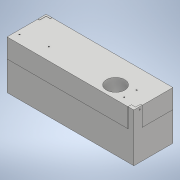
# Autodesk Inventor part: 1руб
Saved by Autodesk Inventor 2020 (Build 240168000, 168)
## iProperties
Created: 2020-02-01
Part Number: 1руб
Material: Типовые
Document SubType Name: Modeling
Designer: Css38
Density: 1 g/cm^3
Appearance: По умолчанию
Author: Css38
Autodesk Inventor part; units mm, degrees
ref_plane "YZ Plane" through (0, 0, 0) normal (1, 0, 0) x (0, 1, 0)
ref_plane "XZ Plane" through (0, 0, 0) normal (0, 1, 0) x (-1, 0, 0)
sketch "Эскиз1" plane through (0, 0, 0) normal (0, 0, 1) x (1, 0, 0)
  line L0 (-76.25, 23.5) -> (76.25, 23.5)
  line L1 (76.25, 23.5) -> (76.25, -23.5)
  line L2 (76.25, -23.5) -> (-76.25, -23.5)
  line L3 (-76.25, -23.5) -> (-76.25, 23.5)
  line L4 (-76.25, 23.5) -> (76.25, -23.5) construction
  line L5 (76.25, 23.5) -> (-76.25, -23.5) construction
  point P0 (0, 0)
  point P1 (0, 0)
  dimension "d35" = 152.5
  dimension "d36" = 47
  constraints: 12 end point, 2 parallel, 1 coincident, 1 horizontal, 1 midpoint, 1 perpendicular
  measures "d35" distance of L1.end L2.end
  measures "d36" distance of L2.end L0.start
extrude "Выдавливание1" add sketch "Эскиз1" along normal blind 30
sketch "Эскиз2" plane through (0, 0, 30) normal (0, 0, 1) x (1, 0, 0)
  line L0 (76.25, 23.5) -> (76.25, -23.5) construction
  line L1 (76.25, -23.5) -> (-76.25, -23.5) construction
  line L2 (-76.25, -23.5) -> (-76.25, 23.5) construction
  line L3 (-76.25, 23.5) -> (76.25, 23.5) construction
  line L4 (74.25, -19.5) -> (51.75, -19.5)
  line L5 (51.75, -19.5) -> (51.75, 3)
  line L6 (51.75, 3) -> (74.25, 3)
  line L7 (74.25, 3) -> (74.25, -19.5)
  point P0 (0, 0)
  dimension "d40" = 22.5
  dimension "d142" = 2
  dimension "d143" = 4
  constraints: 8 end point, 2 parallel, 2 perpendicular, 1 horizontal
  measures "d40" distance of L5.end L6.end
  measures "d142" distance between parallel lines of L0 L7
  measures "d143" distance between parallel lines of L1 L4
extrude "Выдавливание2" cut sketch "Эскиз2" against normal up to next
sketch "Эскиз3" plane through (0, 0, 30) normal (0, 0, 1) x (1, 0, 0)
  line L0 (51.75, 3) -> (51.75, -19.5)
  line L1 (51.75, -19.5) -> (74.25, -19.5)
  line L2 (74.25, -19.5) -> (74.25, 3)
  line L3 (74.25, 3) -> (51.75, 3)
  line L4 (76.25, 23.5) -> (76.25, -23.5) construction
  line L5 (76.25, -23.5) -> (-76.25, -23.5) construction
  line L6 (-76.25, 23.5) -> (76.25, 23.5) construction
  line L7 (76.25, 23.5) -> (-76.25, 23.5) projected
  line L8 (-76.25, 23.5) -> (76.25, 23.5)
  line L9 (76.25, 23.5) -> (76.25, -23.5)
  line L10 (76.25, -23.5) -> (-76.25, -23.5)
  line L11 (-76.25, 23.5) -> (-76.25, 21.5)
  line L12 (-76.25, 23.5) -> (-76.25, -23.5) construction
  line L13 (-76.25, 21.5) -> (6.25, 21.5)
  line L14 (6.25, 21.5) -> (6.25, 3)
  line L15 (6.25, 3) -> (26.25, 3)
  line L16 (26.25, 3) -> (26.25, -19.5)
  line L17 (26.25, -19.5) -> (-76.25, -19.5)
  line L18 (-76.25, -23.5) -> (-76.25, -19.5)
  line L19 (-76.25, -23.5) -> (76.25, -23.5) projected
  line L20 (76.25, -23.5) -> (76.25, 23.5) projected
  line L21 (74.25, -19.5) -> (51.75, -19.5) projected
  line L22 (51.75, -19.5) -> (51.75, 3) projected
  line L23 (51.75, 3) -> (74.25, 3) projected
  line L24 (74.25, 3) -> (74.25, -19.5) projected
  dimension "d50" = 2
  dimension "d63" = 25.5
  dimension "d130" = 20
  constraints: 34 end point, 13 collinear, 4 perpendicular, 2 parallel, 2 point on line
  measures "d50" distance of L6.start L11.end
  measures "d63" distance between parallel lines of L0 L16
  measures "d130" distance of L14.end L15.end
extrude "Выдавливание4" add sketch "Эскиз3" along normal blind 3
sketch "Эскиз4" plane through (0, 0, 33) normal (0, 0, 1) x (1, 0, 0)
  line L0 (51.75, 3) -> (51.75, -19.5) construction
  line L1 (51.75, -19.5) -> (74.25, -19.5) construction
  line L2 (74.25, -19.5) -> (74.25, 3) construction
  line L3 (74.25, 3) -> (51.75, 3) construction
  line L4 (76.25, 23.5) -> (76.25, -23.5) projected
  line L5 (76.25, -23.5) -> (-76.25, -23.5) projected
  line L6 (-76.25, -23.5) -> (-76.25, -19.5) projected
  line L7 (-76.25, -19.5) -> (26.25, -19.5) projected
  line L8 (26.25, -19.5) -> (26.25, 3) projected
  line L9 (26.25, 3) -> (6.25, 3) projected
  line L10 (6.25, 3) -> (6.25, 21.5) projected
  line L11 (6.25, 21.5) -> (-76.25, 21.5) projected
  line L12 (-76.25, 21.5) -> (-76.25, 23.5) projected
  line L13 (-76.25, 23.5) -> (76.25, 23.5) projected
  line L14 (26.25, -19.5) -> (26.25, 3) projected
  line L15 (26.25, 3) -> (51.75, 3) construction
  line L16 (51.75, 3) -> (51.75, -19.5) projected
  line L17 (51.75, -19.5) -> (26.25, -19.5) construction
  circle A0 centre (39, -8.25) radius 11
  line L18 (39, -8.25) -> (39, 3) construction
  line L19 (39, -8.25) -> (39, -19.5) construction
  line L20 (51.75, -19.5) -> (51.75, 3) construction
  line L21 (39, -8.25) -> (26.25, -8.25) construction
  line L22 (39, -8.25) -> (51.75, -8.25) construction
  point P0 (0, 0)
  dimension "d55" = 22
  constraints: 12 end point, 4 midpoint, 3 perpendicular, 2 collinear, 1 centre point, 1 point on line, 1 other
  measures "d55" diameter of A0
extrude "Выдавливание7" add sketch "Эскиз4" along normal blind 25
sketch "Эскиз6" plane through (26.25, -19.5, 30) normal (-1, 0, 0) x (0, 0, 1)
  line L0 (3, 0.25) -> (3, 22.25) construction
  line L1 (0, 22.5) -> (28, 22.5) projected
  line L2 (0, 0) -> (28, 0) projected
  line L3 (3, 22.5) -> (5, 22.5)
  line L4 (5, 22.5) -> (5, 0)
  line L5 (5, 0) -> (3, 0)
  line L6 (3, 0) -> (3, 22.5)
  point P0 (-30, 19.5)
  dimension "d66" = 2
  constraints: 8 end point, 2 parallel, 2 point on line, 1 collinear, 1 horizontal, 1 perpendicular
  measures "d66" distance of L4.end L5.end
extrude "Выдавливание8" cut sketch "Эскиз6" against normal up to surface (48 mm away) from surface at 0
sketch "Эскиз7" plane through (0, 0, 58) normal (0, 0, 1) x (1, 0, 0)
  line L0 (76.25, -23.5) -> (-76.25, -23.5) projected
  line L1 (-76.25, 23.5) -> (76.25, 23.5) projected
  line L2 (76.25, -23.5) -> (-76.25, -23.5)
  line L3 (-76.25, -23.5) -> (-76.25, 23.5)
  line L4 (-76.25, 23.5) -> (76.25, 23.5)
  line L5 (76.25, 23.5) -> (76.25, -23.5)
  circle A0 centre (39, -8.25) radius 11 projected
  point P0 (0, 0)
  constraints: 8 end point, 2 parallel, 1 horizontal, 1 perpendicular
extrude "Выдавливание9" add sketch "Эскиз7" against normal blind 17.15
ref_plane "РабПлоскость1" through (26.25, 3, 35) normal (0, 0, -1) x (-1, 0, 0)
split body "Разделение1" result two bodies by plane through (26.25, 3, 35) normal (0, 0, -1) first body at (-33.5833, 1, 0.5)
sketch "Эскиз22" plane through (0, 0, 30) normal (0, 0, 1) x (1, 0, 0)
  line L0 (-76.25, -19.5) -> (26.25, -19.5) construction
  line L1 (26.25, -19.5) -> (26.25, 3) construction
  line L2 (26.25, 3) -> (6.25, 3) construction
  line L3 (6.25, 3) -> (6.25, 21.5) construction
  line L4 (6.25, 21.5) -> (-76.25, 21.5) construction
  line L5 (-76.25, -19.5) -> (-76.25, 21.5) construction
  line L6 (-76.25, -23.5) -> (-76.25, -19.5) construction
  line L7 (76.25, -23.5) -> (-76.25, -23.5) construction
  line L8 (76.25, 23.5) -> (76.25, -23.5) construction
  line L9 (-76.25, 23.5) -> (76.25, 23.5) construction
  line L10 (74.25, 3) -> (51.75, 3) construction
  line L11 (51.75, 3) -> (51.75, -19.5) construction
  line L12 (51.75, -19.5) -> (74.25, -19.5) construction
  line L13 (74.25, -19.5) -> (74.25, 3) construction
  line L14 (-76.25, -19.5) -> (-43.25, -19.5)
  line L15 (-43.25, -19.5) -> (-43.25, -7)
  line L16 (-43.25, -7) -> (-76.25, -7)
  line L17 (-76.25, -7) -> (-76.25, -19.5)
  line L18 (-76.25, 21.5) -> (-76.25, 23.5) projected
  point P0 (0, 0)
  dimension "d144" = 33
  dimension "d145" = 12.5
  constraints: 8 end point, 2 parallel, 1 horizontal, 1 perpendicular
  measures "d144" distance of L16.end L15.end
  measures "d145" distance of L15.end L14.end
extrude "Выдавливание26" cut sketch "Эскиз22" against normal blind 28 bodies 2
sketch "Эскиз23" plane through (0, 0, 2) normal (0, 0, 1) x (1, 0, 0)
  line L0 (76.25, 23.5) -> (76.25, -23.5) construction
  line L1 (76.25, -23.5) -> (-76.25, -23.5) construction
  line L2 (-76.25, -23.5) -> (-76.25, -19.5) construction
  line L3 (-76.25, -19.5) -> (-76.25, -7) construction
  line L4 (-43.25, -7) -> (-76.25, -7) construction
  line L5 (-43.25, -19.5) -> (-43.25, -7) construction
  line L6 (-76.25, -19.5) -> (-43.25, -19.5) construction
  line L7 (-76.25, 23.5) -> (76.25, 23.5) construction
  line L8 (-76.25, -7) -> (-76.25, 23.5) construction
  line L9 (74.25, 3) -> (51.75, 3) construction
  line L10 (51.75, 3) -> (51.75, -19.5) construction
  line L11 (51.75, -19.5) -> (74.25, -19.5) construction
  line L12 (74.25, -19.5) -> (74.25, 3) construction
  line L13 (-43.25, -19.5) -> (-47.75, -19.5)
  line L14 (-47.75, -19.5) -> (-47.75, -7)
  line L15 (-47.75, -7) -> (-43.25, -7)
  line L16 (-43.25, -7) -> (-43.25, -19.5)
  point P0 (0, 0)
  dimension "d148" = 4.5
  constraints: 8 end point, 2 parallel, 1 horizontal, 1 perpendicular, 1 point on line
  measures "d148" distance of L14.end L15.end
extrude "Выдавливание27" add sketch "Эскиз23" along normal blind 18 bodies 2
sketch "Эскиз24" plane through (0, 0, 20) normal (0, 0, 1) x (1, 0, 0)
  line L0 (76.25, 23.5) -> (76.25, -23.5) construction
  line L1 (76.25, -23.5) -> (-76.25, -23.5) construction
  line L2 (-76.25, -23.5) -> (-76.25, -19.5) construction
  line L3 (-76.25, -19.5) -> (-47.75, -19.5) construction
  line L4 (-47.75, -19.5) -> (-47.75, -7) construction
  line L5 (-43.25, -7) -> (-47.75, -7) construction
  line L6 (-43.25, -19.5) -> (-43.25, -7) construction
  line L7 (-47.75, -19.5) -> (-43.25, -19.5) construction
  line L8 (-76.25, 23.5) -> (76.25, 23.5) construction
  line L9 (-76.25, -7) -> (-76.25, 23.5) construction
  line L10 (-47.75, -7) -> (-76.25, -7) construction
  line L11 (74.25, 3) -> (51.75, 3) construction
  line L12 (51.75, 3) -> (51.75, -19.5) construction
  line L13 (51.75, -19.5) -> (74.25, -19.5) construction
  line L14 (74.25, -19.5) -> (74.25, 3) construction
  line L15 (-76.25, -7) -> (-47.75, -7) construction
  line L16 (-43.25, -19.5) -> (-47.75, -7) construction
  line L17 (-47.75, -19.5) -> (-47.75, -7) construction
  line L18 (-47.75, -7) -> (-47.75, -19.5) construction
  line L19 (-47.75, -19.5) -> (-43.25, -7) construction
  circle A0 centre (-45.5, -13.25) radius 0.75
  point P0 (0, 0)
  dimension "d151" = 1.5
  constraints: 6 end point, 1 centre point, 1 collinear, 1 midpoint
  measures "d151" diameter of A0
extrude "Выдавливание28" cut sketch "Эскиз24" against normal blind 3 bodies 2
sketch "Эскиз25" plane through (0, 0, 30) normal (0, 0, 1) x (1, 0, 0)
  line L0 (76.25, 23.5) -> (76.25, -23.5) construction
  line L1 (76.25, -23.5) -> (-76.25, -23.5) construction
  line L2 (-76.25, -23.5) -> (-76.25, -19.5) construction
  line L3 (-76.25, -19.5) -> (-43.25, -19.5) construction
  line L4 (-43.25, -19.5) -> (26.25, -19.5) construction
  line L5 (26.25, -19.5) -> (26.25, 3) construction
  line L6 (26.25, 3) -> (6.25, 3) construction
  line L7 (6.25, 3) -> (6.25, 21.5) construction
  line L8 (6.25, 21.5) -> (-76.25, 21.5) construction
  line L9 (-76.25, -7) -> (-76.25, 21.5) construction
  line L10 (-43.25, -7) -> (-76.25, -7) construction
  line L11 (-43.25, -19.5) -> (-43.25, -7) construction
  line L12 (-76.25, 23.5) -> (76.25, 23.5) construction
  line L13 (74.25, 3) -> (51.75, 3) construction
  line L14 (51.75, 3) -> (51.75, -19.5) construction
  line L15 (51.75, -19.5) -> (74.25, -19.5) construction
  line L16 (74.25, -19.5) -> (74.25, 3) construction
  line L17 (-76.25, -19.5) -> (-76.25, -7) construction
  line L18 (51.75, 3) -> (51.75, -19.5) construction
  line L19 (27.3887, -8.25) -> (-21.6113, -8.25)
  line L20 (-65.25, -13.25) -> (-45.6782, 15.7663)
  line L21 (-43.25, -7) -> (-43.25, -19.5) construction
  line L22 (-45.6782, 15.7663) -> (-21.6113, -8.25)
  line L23 (-76.25, 21.5) -> (-76.25, 23.5) projected
  point P0 (0, 0)
  point P1 (-43.25, -13.25)
  point P2 (51.75, -8.25)
  dimension "d154" = 11
  dimension "d155" = 49
  dimension "d156" = 35
  dimension "d159" = 34
  dimension "d164" = 56
  constraints: 6 end point, 2 midpoint, 1 horizontal, 1 horizontal alignment, 1 point on line
  measures "d154" distance from line of L17 L20.start
  measures "d155" distance of L19.start L19.end
  measures "d156" distance of L20.start L20.end
  measures "d159" distance of L20.end L19.end
  measures "d164" angle of L4 L20
sketch "Эскиз20" plane through (0, 0, 58) normal (0, 0, 1) x (1, 0, 0)
  line L0 (-76.25, -23.5) -> (76.25, -23.5) construction
  line L1 (-76.25, 23.5) -> (-76.25, -23.5) construction
  line L2 (62, -23.5) -> (-46, -23.5) construction
  line L3 (-46, -23.5) -> (-46, 6.5) construction
  line L4 (-46, 6.5) -> (-36, 6.5) construction
  line L5 (76.25, -23.5) -> (-76.25, -23.5) construction
  line L6 (0, -32.9) -> (0, 32.9) construction
  line L7 (62, 6.5) -> (62, -8.5) construction
  circle A0 centre (39, -8.25) radius 11 construction
  line L8 (-76.25, -23.5) -> (76.25, -23.5) construction
  circle A1 centre (-71.25, -13.5) radius 0.5
  line L9 (-36, 6.5) -> (-36, -23.5) construction
  line L10 (-76.25, -23.5) -> (76.25, -23.5) construction
  line L11 (52, 6.5) -> (52, -23.5) construction
  line L12 (-36, 6.5) -> (52, 6.5) construction
  line L13 (52, 6.5) -> (62, 6.5) construction
  line L14 (-46, 6.5) -> (-36, -23.5) construction
  line L15 (-36, 6.5) -> (-46, -23.5) construction
  line L16 (62, 6.5) -> (52, -8.5) construction
  line L17 (52, -8.5) -> (62, -23.5) construction
  line L18 (52, -23.5) -> (62, -8.5) construction
  line L19 (52, 6.5) -> (62, -8.5) construction
  line L20 (62, -8.5) -> (62, -23.5) construction
  circle A2 centre (-41, -8.5) radius 0.5
  circle A3 centre (57, -1) radius 0.5
  circle A4 centre (57, -16) radius 0.5
  point P0 (0, 0)
  point P1 (-41, -8.5)
  dimension "d136" = 30
  dimension "d167" = 10
  dimension "d168" = 5
  dimension "d169" = 10
  dimension "d170" = 1
  dimension "d241" = 108
  dimension "d242" = 2
  constraints: 30 end point, 6 midpoint, 4 centre point, 4 collinear, 3 equal radius, 3 perpendicular, 3 point on line, 2 horizontal alignment, 2 parallel, 1 horizontal
  measures "d136" distance between parallel lines of L0 L4
  measures "d167" distance from line of L0 A1.centre
  measures "d168" distance from line of L1 A1.centre
  measures "d169" distance between parallel lines of L3 L9
  measures "d170" diameter of A2
  measures "d241" distance between parallel lines of L7 L3
  measures "d242" distance edge to line of A0 L11
hole "Отверстие1" at (-71.25, -13.5, 58) at (-41, -8.5, 58) at (57, -16, 58) at (57, -1, 58) direction (0, 0, -1) diameter 1 depth 5 tip angle 118 countersink diameter 1.5 countersink angle 90 bodies 3
sketch "Эскиз28" plane through (0, 0, 30) normal (0, 0, 1) x (1, 0, 0)
  line L0 (-76.25, -23.5) -> (-76.25, -19.5) construction
  line L1 (-76.25, -19.5) -> (-43.25, -19.5) construction
  line L2 (-43.25, -19.5) -> (-43.25, -7) construction
  line L3 (-43.25, -7) -> (-76.25, -7) construction
  line L4 (-76.25, -7) -> (-76.25, 21.5) construction
  line L5 (-76.25, 21.5) -> (-76.25, 23.5) construction
  line L6 (-76.25, 23.5) -> (76.25, 23.5) construction
  line L7 (76.25, 23.5) -> (76.25, -23.5) construction
  line L8 (76.25, -23.5) -> (-76.25, -23.5) construction
  line L9 (-43.25, -19.5) -> (26.25, -19.5) construction
  line L10 (26.25, -19.5) -> (26.25, 3) construction
  line L11 (26.25, 3) -> (6.25, 3) construction
  line L12 (6.25, 3) -> (6.25, 21.5) construction
  line L13 (6.25, 21.5) -> (-76.25, 21.5) construction
  line L14 (74.25, 3) -> (51.75, 3) construction
  line L15 (51.75, 3) -> (51.75, -19.5) construction
  line L16 (51.75, -19.5) -> (74.25, -19.5) construction
  line L17 (74.25, -19.5) -> (74.25, 3) construction
  line L18 (-76.25, 23.5) -> (76.25, 23.5) construction
  line L19 (-76.25, 23.5) -> (-76.25, 13.5)
  line L20 (-76.25, -23.5) -> (-76.25, 23.5) construction
  line L21 (-76.25, 13.5) -> (-74.25, 13.5)
  line L22 (-74.25, 13.5) -> (-74.25, 21.5)
  line L23 (-76.25, 23.5) -> (-69.25, 23.5)
  line L24 (-69.25, 23.5) -> (-69.25, 21.5)
  line L25 (-69.25, 21.5) -> (-74.25, 21.5)
  line L26 (76.25, -23.5) -> (-76.25, -23.5) construction
  line L27 (76.25, -23.5) -> (76.25, -13.5)
  line L28 (76.25, 23.5) -> (76.25, -23.5) construction
  line L29 (76.25, -13.5) -> (74.25, -13.5)
  line L30 (74.25, -19.5) -> (74.25, 3) construction
  line L31 (74.25, -13.5) -> (74.25, -19.5)
  line L32 (74.25, -19.5) -> (69.25, -19.5)
  line L33 (51.75, -19.5) -> (74.25, -19.5) construction
  line L34 (69.25, -19.5) -> (69.25, -23.5)
  line L35 (69.25, -23.5) -> (76.25, -23.5)
  point P0 (0, 0)
  dimension "d199" = 10
  dimension "d200" = 2
  dimension "d201" = 7
  dimension "d202" = 10
  dimension "d203" = 5
  constraints: 24 end point, 8 point on line, 6 perpendicular, 2 collinear
  measures "d199" distance of L5.end L19.end
  measures "d200" distance of L19.end L21.end
  measures "d201" distance of L5.end L23.end
  measures "d202" distance of L7.end L27.end
  measures "d203" distance of L16.end L32.end
extrude "Выдавливание31" add sketch "Эскиз28" along normal blind 28.1 bodies 2
sketch "Эскиз29" plane through (0, 0, 58) normal (0, 0, 1) x (1, 0, 0)
  line L0 (69.25, -23.5) -> (69.25, -19.5) construction
  line L1 (69.25, -19.5) -> (74.25, -19.5) construction
  line L2 (74.25, -19.5) -> (74.25, -13.5) construction
  line L3 (74.25, -13.5) -> (76.25, -13.5) construction
  line L4 (76.25, -13.5) -> (76.25, -23.5) construction
  line L5 (76.25, -23.5) -> (69.25, -23.5) construction
  line L6 (-74.25, 13.5) -> (-76.25, 13.5) construction
  line L7 (-76.25, 13.5) -> (-76.25, 23.5) construction
  line L8 (-76.25, 23.5) -> (-69.25, 23.5) construction
  line L9 (-69.25, 23.5) -> (-69.25, 21.5) construction
  line L10 (-69.25, 21.5) -> (-74.25, 21.5) construction
  line L11 (-74.25, 21.5) -> (-74.25, 13.5) construction
  circle A0 centre (57, -16) radius 0.75 construction
  circle A1 centre (-71.25, -13.5) radius 0.75 construction
  circle A2 centre (-41, -8.5) radius 0.75 construction
  circle A3 centre (57, -1) radius 0.75 construction
  line L12 (-76.25, -23.5) -> (-76.25, 23.5) construction
  line L13 (-76.25, 23.5) -> (76.25, 23.5) construction
  line L14 (76.25, 23.5) -> (76.25, -23.5) construction
  line L15 (76.25, -23.5) -> (-76.25, -23.5) construction
  circle A4 centre (39, -8.25) radius 11 construction
  line L16 (-74.15, 13.4) -> (-76.35, 13.4)
  line L17 (-76.35, 13.4) -> (-76.35, 23.6)
  line L18 (-76.35, 23.6) -> (-69.15, 23.6)
  line L19 (-69.15, 23.6) -> (-69.15, 21.4)
  line L20 (-69.15, 21.4) -> (-74.15, 21.4)
  line L21 (-74.15, 21.4) -> (-74.15, 13.4)
  line L22 (74.15, -13.4) -> (74.15, -19.4)
  line L23 (74.15, -19.4) -> (69.15, -19.4)
  line L24 (69.15, -19.4) -> (69.15, -23.6)
  line L25 (69.15, -23.6) -> (76.35, -23.6)
  line L26 (76.35, -23.6) -> (76.35, -13.4)
  line L27 (76.35, -13.4) -> (74.15, -13.4)
  point P0 (0, 0)
  dimension "d206" = 0.1
  dimension "d207" = 0.1
  constraints: 24 end point, 10 other
  measures "d206" distance between parallel lines of L11 L21
  measures "d207" distance between parallel lines of L2 L22
extrude "Выдавливание32" cut sketch "Эскиз29" against normal through all bodies 3
sketch "Эскиз30" plane through (76.25, -23.5, 0) normal (1, 0, 0) x (0, 0, -1)
  line L0 (0, 4) -> (-58.1, 4) construction
  line L1 (-58.1, 4) -> (-52.1, 4) construction
  line L2 (-52.1, 4) -> (-52.1, 10) construction
  line L3 (-52.1, 10) -> (-58.1, 10) construction
  line L4 (-58.1, 10) -> (-58.1, 4) construction
  line L5 (-35, 10) -> (-58.1, 10) construction
  line L6 (-58.1, 4) -> (-52.1, 10) construction
  line L7 (-58.1, 10) -> (-58.1, 4) construction
  line L8 (-52.1, 4) -> (-58.1, 10) construction
  circle A0 centre (-55.1, 7) radius 0.5
  point P0 (0, 23.5)
  dimension "d210" = 1
  constraints: 12 end point, 3 perpendicular, 2 parallel, 1 centre point, 1 collinear, 1 horizontal, 1 midpoint
  measures "d210" diameter of A0
hole "Отверстие4" at (76.25, -16.5, 55.1) direction (-1, 0, 0) diameter 1 end through all countersink diameter 1.5 countersink angle 90 bodies 2
sketch "Эскиз31" plane through (-76.25, -23.5, 0) normal (-1, 0, 0) x (0, 0, 1)
  line L0 (58.1, 45) -> (30, 45) construction
  circle A0 centre (55.1, 7) radius 0.5 construction
  line L1 (30, 37) -> (58.1, 37) construction
  line L2 (58.1, 37) -> (58.1, 45) construction
  line L3 (58.1, 45) -> (30, 37) construction
  line L4 (30, 26.5) -> (30, 45) construction
  line L5 (30, 45) -> (58.1, 37) construction
  circle A1 centre (55.1, 41) radius 0.5
  point P0 (0, 23.5)
  point P1 (44.05, 41)
  constraints: 4 end point, 1 centre point, 1 equal radius, 1 horizontal alignment, 1 midpoint, 1 vertical alignment
hole "Отверстие5" at (-76.25, 17.5, 55.1) direction (1, 0, 0) diameter 1 end through all countersink diameter 1.5 countersink angle 90 bodies 2
sketch "Эскиз32" plane through (74.15, -19.4, 58) normal (1, 0, 0) x (0, 0, -1)
  circle A0 centre (2.9, 2.9) radius 0.5 construction
  circle A1 centre (3, 2.9) radius 0.5
  point P0 (58, 19.4)
  dimension "d225" = 0.1
  constraints: 1 centre point, 1 equal radius, 1 horizontal alignment
  measures "d225" distance of A0.centre A1.centre
hole "Отверстие6" at (74.15, -16.5, 55) direction (-1, 0, 0) diameter 1 depth 5 tip angle 118 countersink diameter 1.5 countersink angle 90 bodies 3
sketch "Эскиз33" plane through (-74.15, 13.4, 58) normal (-1, 0, 0) x (0, 0, 1)
  circle A0 centre (-2.9, 4.1) radius 0.5 construction
  circle A1 centre (-3, 4.1) radius 0.5
  point P0 (-58, -13.4)
  dimension "d233" = 0.1
  constraints: 1 centre point, 1 equal radius, 1 horizontal alignment
  measures "d233" distance of A0.centre A1.centre
hole "Отверстие7" at (-74.15, 17.5, 55) direction (1, 0, 0) diameter 1 depth 5 tip angle 118 countersink diameter 1.5 countersink angle 90 bodies 3
